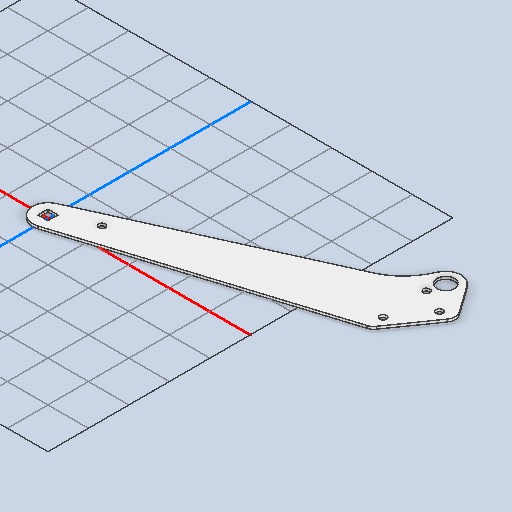
# Autodesk Inventor part: Gusset
Saved by Autodesk Inventor 2026 (Build 300175000, 175)
## iProperties
Created: 2025-04-12
Part Number: Gusset
Material: Acetal Resin, White
Document SubType Name: Modeling
Designer: avere
Density: 1.425 g/cm^3
Appearance: Smooth - White
Author: avere
Autodesk Inventor part; units mm, degrees
ref_plane "YZ Plane" through (0, 0, 0) normal (1, 0, 0) x (0, 1, 0)
ref_plane "XZ Plane" through (0, 0, 0) normal (0, 1, 0) x (-1, 0, 0)
ref_plane "XY Plane" through (0, 0, 0) normal (0, 0, 1) x (1, 0, 0)
sketch "main" plane through (0, 0, 0) normal (0, 0, 1) x (1, 0, 0)
  arc A0 (-76.9765, 33.0075) -> (-80.2841, 30.5888) centre (-75.0825, 26.9465) ccw
  circle A1 centre (-77.4831, 23.5181) radius 2.1844
  circle A2 centre (-76.8428, -4.4337) radius 2.1844
  arc A3 (-57.2294, -80.4633) -> (-56.4581, -83.5168) centre (-56.6485, -81.9407) ccw
  circle A4 centre (-92.052, 2.7116) radius 2.1844
  circle A5 centre (-78.8735, -14.4473) radius 5.5563
  line L0 (-80.2841, 30.5888) -> (-98.7239, 4.254)
  arc A6 (-98.7239, 4.254) -> (-98.6909, -3.0772) centre (-93.5223, 0.6117) ccw
  arc A7 (-86.6264, -19.9807) -> (-70.0421, -18.0155) centre (-78.8735, -14.4473) ccw
  line L1 (-98.6909, -3.0772) -> (-86.6264, -19.9807)
  arc A8 (87.0859, 64.3881) -> (80.3336, 82.1644) centre (83.1745, 73.0729) ccw
  line L2 (86.3241, 76.2225) -> (80.0249, 76.2225)
  line L3 (80.0249, 76.2225) -> (80.0249, 69.9233)
  line L4 (80.0249, 69.9233) -> (86.3241, 69.9233)
  line L5 (86.3241, 69.9233) -> (86.3241, 76.2225)
  line L6 (86.3241, 76.2225) -> (80.0249, 69.9233) construction
  line L7 (80.0249, 76.2225) -> (86.3241, 69.9233) construction
  circle A9 centre (60.3149, 62.0006) radius 2.1844
  line L8 (87.0859, 64.3881) -> (-50.3044, 2.5112)
  arc A10 (-50.3044, 2.5112) -> (-70.0421, -18.0155) centre (-34.6127, -32.3302) ccw
  line L9 (80.3336, 82.1644) -> (-76.9765, 33.0075)
  point P0 (-51.4681, 8.9463)
  point P1 (-79.4455, 31.7864)
  point P2 (-101.2988, 0.5767)
  dimension "d4" = 11.1125
  dimension "d5" = 19.05
  dimension "d6" = 19.05
  dimension "d7" = 38.1
  dimension "d8" = 4.3688
  dimension "d9" = 6.35
  dimension "d10" = 25.4
  dimension "d11" = 6.35
  dimension "d13" = 4.3688
  dimension "d20" = 6.2992
  dimension "d21" = 6.2992
  dimension "d24" = 4.3688
  dimension "d25" = 25.4
  measures "d4" diameter of A5
  measures "d5" diameter of A7
  measures "d6" diameter of A8
  measures "d7" distance of point (-79.446, 31.786) point (-101.299, 0.577)
  measures "d8" diameter of A1
  measures "d9" distance from line of L0 A1.centre
  measures "d10" distance of A1.centre A4.centre
  measures "d11" radius of A0
  measures "d13" diameter of A2
  measures "d20" distance of L4.end L3.end
  measures "d21" distance of L3.end L2.end
  measures "d24" diameter of A9
  measures "d25" distance of A8.centre A9.centre
sketch "Sketch1" plane through (0, 0, 0) normal (0, 1, 0) x (-1, 0, 0)
  arc A0 (-160.151, -40.0654) -> (-163.4586, -42.4842) centre (-158.257, -46.1264) ccw
  circle A1 centre (-160.6577, -49.5549) radius 2.1844
  circle A2 centre (-160.0174, -77.5067) radius 2.1844
  arc A3 (-140.4039, -153.5363) -> (-139.6326, -156.5897) centre (-139.823, -155.0137) ccw
  circle A4 centre (-175.2265, -70.3613) radius 2.1844
  circle A5 centre (-162.048, -87.5202) radius 5.5563
  line L0 (-163.4586, -42.4842) -> (-181.8985, -68.819)
  arc A6 (-181.8985, -68.819) -> (-181.8654, -76.1501) centre (-176.6968, -72.4612) ccw
  arc A7 (-169.8009, -93.0537) -> (-153.2166, -91.0884) centre (-162.048, -87.5202) ccw
  line L1 (-181.8654, -76.1501) -> (-169.8009, -93.0537)
  arc A8 (3.9114, -8.6848) -> (-2.8409, 9.0915) centre (0, 0) ccw
  line L2 (3.1496, 3.1496) -> (-3.1496, 3.1496)
  line L3 (-3.1496, 3.1496) -> (-3.1496, -3.1496)
  line L4 (-3.1496, -3.1496) -> (3.1496, -3.1496)
  line L5 (3.1496, -3.1496) -> (3.1496, 3.1496)
  line L6 (3.1496, 3.1496) -> (-3.1496, -3.1496) construction
  line L7 (-3.1496, 3.1496) -> (3.1496, -3.1496) construction
  circle A9 centre (-22.8596, -11.0724) radius 2.1844
  line L8 (3.9114, -8.6848) -> (-133.4789, -70.5617)
  arc A10 (-133.4789, -70.5617) -> (-153.2166, -91.0884) centre (-117.7873, -105.4032) ccw
  line L9 (-2.8409, 9.0915) -> (-160.151, -40.0654)
  point P0 (0, 0)
extrude "Extrusion1" add sketch "Sketch1" along normal blind 1.5875
body "Solid1"
